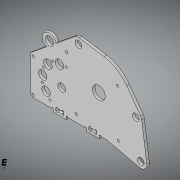
# Autodesk Inventor part: 新型４アームフレーム新
Saved by Autodesk Inventor 2019 (Build 230136000, 136)
## iProperties
Created: 2019-09-30
Part Number: 新型４アームフレーム新
Material: 一般
Document SubType Name: Modeling
Designer: tanjihayato
Density: 1 g/cm^3
Appearance: 既定
Author: tanjihayato
Autodesk Inventor part; units mm, degrees
ref_plane "YZ Plane" through (0, 0, 0) normal (1, 0, 0) x (0, 1, 0)
ref_plane "XZ Plane" through (0, 0, 0) normal (0, 1, 0) x (-1, 0, 0)
ref_plane "XY Plane" through (0, 0, 0) normal (0, 0, 1) x (1, 0, 0)
sketch "スケッチ1" plane through (0, 0, 0) normal (0, 0, 1) x (1, 0, 0)
  circle A0 centre (-22.9427, -32.8237) radius 14
  circle A1 centre (5.0573, -32.8237) radius 14
  line L0 (-174.7493, -46.8237) -> (173.7138, -46.8237)
  line L1 (-168.9427, 85.6498) -> (-168.9427, -143.3841)
  line L2 (181.0573, 70.1234) -> (181.0573, -176.3692)
  line L3 (-68.9427, 93.6608) -> (-68.9427, -144.401)
  circle A2 centre (-138.9427, -9.8237) radius 4.5
  circle A3 centre (-32.6636, -19.9769) radius 20.05
  circle A4 centre (-50.9427, -32.8237) radius 14
  circle A5 centre (-48.8152, -4.5402) radius 14
  circle A6 centre (-32.6636, -19.9769) radius 9.0359
  circle A7 centre (10.5145, -3.7237) radius 37.1
  circle A8 centre (-48.8152, -4.5402) radius 2.292
  circle A9 centre (-48.8152, -4.5402) radius 2.792
  circle A10 centre (10.5145, -3.7237) radius 39.1
  circle A11 centre (53.6032, -6.8237) radius 33.1
  circle A12 centre (53.6032, -6.8237) radius 35.1
  line L4 (-120.6193, -91.8237) -> (100.4081, -91.8237)
  circle A13 centre (10.5145, -3.7237) radius 10.1
  circle A14 centre (10.5145, -3.7237) radius 12.1
  circle A15 centre (-32.6636, -19.9769) radius 20.55
  line L5 (53.6032, -6.8237) -> (32.39, 14.3895)
  line L6 (53.6032, -6.8237) -> (97.5006, -47.7262)
  line L7 (97.5006, -47.7262) -> (57.2048, -10.293)
  line L8 (57.2048, -10.293) -> (32.39, 14.3895)
  circle A16 centre (32.39, 14.3895) radius 1.5
  circle A17 centre (32.39, 14.3895) radius 4.5
  circle A18 centre (-54.9427, -18.301) radius 14
  circle A19 centre (-35.3456, 2.2036) radius 14
  circle A20 centre (-50.9427, -32.8237) radius 5
  circle A21 centre (-54.9427, -18.301) radius 5
  circle A22 centre (-48.8152, -4.5402) radius 5
  circle A23 centre (-35.3456, 2.2036) radius 5
  circle A24 centre (-32.6636, -19.9769) radius 22.342 construction
  line L9 (-43.4189, -43.5289) -> (-55.5427, -26.2785) construction
  line L10 (-55.5427, -26.2785) -> (-54.3426, -10.3236) construction
  line L11 (-54.3426, -10.3236) -> (-43.2878, 1.2432) construction
  line L12 (-43.2878, 1.2432) -> (-22.1495, 3.7992) construction
  circle A25 centre (-35.3456, 2.2036) radius 8
  circle A26 centre (-48.8152, -4.5402) radius 8
  circle A27 centre (-54.9427, -18.301) radius 8
  circle A28 centre (-50.9427, -32.8237) radius 8
  circle A29 centre (-46.3426, -39.3689) radius 1.3
  circle A30 centre (-55.5427, -26.2785) radius 1.3
  circle A31 centre (-54.3426, -10.3236) radius 1.3
  circle A32 centre (-43.2878, 1.2432) radius 1.3
  circle A33 centre (-27.4035, 3.1639) radius 1.3
  circle A34 centre (-35.3456, 2.2036) radius 5.5 construction
  line L13 (-89.4402, -42.8237) -> (131.6872, -42.8237)
  circle A35 centre (53.6032, -6.8237) radius 3
  circle A36 centre (97.5006, -47.7262) radius 7.025
  circle A37 centre (97.5006, -47.7262) radius 10.025
  circle A38 centre (57.2048, -10.293) radius 5
  line L14 (60.2589, -6.3341) -> (103.6241, -39.7887)
  line L15 (90.035, -54.4169) -> (53.4813, -13.63)
  point P0 (0, 0)
  point P1 (0, 0)
  point P2 (0, 0)
  dimension "d0" = 350
  dimension "d1" = 100
  dimension "d2" = 30
  dimension "d3" = 40.1
  dimension "d4" = 28
  dimension "d5" = 28
  dimension "d6" = 22.342
  dimension "d7" = 22.342
  dimension "d9" = 74.2
  dimension "d10" = 0.5
  dimension "d11" = 2
  dimension "d13" = 66.2
  dimension "d14" = 2
  dimension "d15" = 45
  dimension "d16" = 85
  dimension "d17" = 2
  dimension "d18" = 0.5
  dimension "d19" = 30
  dimension "d20" = 60
  dimension "d21" = 55
  dimension "d22" = 35
  dimension "d23" = 45
  dimension "d24" = 3
  dimension "d25" = 3
  dimension "d26" = 28
  dimension "d27" = 28
  dimension "d28" = 22.342
  dimension "d29" = 22.342
  dimension "d30" = 10
  dimension "d31" = 10
  dimension "d32" = 10
  dimension "d33" = 10
  dimension "d34" = 3
  dimension "d35" = 3
  dimension "d36" = 3
  dimension "d37" = 3
  dimension "d38" = 2.6
  dimension "d39" = 2.6
  dimension "d40" = 2.6
  dimension "d41" = 2.6
  dimension "d42" = 2.6
  dimension "d43" = 11
  dimension "d44" = 20.2
  dimension "d45" = 4
  dimension "d46" = 6
  dimension "d48" = 46.1359
  dimension "d60" = 14.05
  dimension "d61" = 3
  dimension "d62" = 10
  constraints: 38 centre point, 32 end point, 14 coincident, 12 point on circle, 10 tangent, 7 point on line, 4 vertical, 3 horizontal, 2 midpoint, 1 equal radius, 9 other
  measures "d0" distance between parallel lines of L2 L1
  measures "d1" distance between parallel lines of L1 L3
  measures "d2" distance from line of L1 A2.centre
  measures "d3" diameter of A3
  measures "d4" diameter of A4
  measures "d5" diameter of A5
  measures "d6" distance of A5.centre A3.centre
  measures "d7" distance of A4.centre A3.centre
  measures "d9" diameter of A7
  measures "d10" radial gap between concentric circles of A8 A9
  measures "d11" radial gap between concentric circles of A7 A10
  measures "d13" diameter of A11
  measures "d14" radial gap between concentric circles of A11 A12
  measures "d15" distance between parallel lines of L4 L0
  measures "d16" distance from line of L4 L5.start
  measures "d17" radial gap between concentric circles of A13 A14
  measures "d18" radial gap between concentric circles of A3 A15
  measures "d19" distance of L5.start L5.end
  measures "d20" distance of L5.start L6.end
  measures "d21" distance of L6.end L7.end
  measures "d22" distance of L7.end L5.end
  measures "d23" angle of L0 L5
  measures "d24" diameter of A16
  measures "d25" radial gap between concentric circles of A16 A17
  measures "d26" diameter of A18
  measures "d27" diameter of A19
  measures "d28" distance of A3.centre A19.centre
  measures "d29" distance of A3.centre A18.centre
  measures "d30" diameter of A20
  measures "d31" diameter of A21
  measures "d32" diameter of A22
  measures "d33" diameter of A23
  measures "d34" radial gap between concentric circles of A23 A25
  measures "d35" radial gap between concentric circles of A22 A26
  measures "d36" radial gap between concentric circles of A21 A27
  measures "d37" radial gap between concentric circles of A20 A28
  measures "d38" diameter of A29
  measures "d39" diameter of A30
  measures "d40" diameter of A31
  measures "d41" diameter of A32
  measures "d42" diameter of A33
  measures "d43" diameter of A34
  measures "d44" diameter of A13
  measures "d45" distance between parallel lines of L0 L13
  measures "d46" diameter of A35
  measures "d48" distance of A3.centre A13.centre
  measures "d60" diameter of A36
  measures "d61" radial gap between concentric circles of A36 A37
  measures "d62" diameter of A38
sketch "スケッチ2" plane through (0, 0, 0) normal (0, 0, 1) x (1, 0, 0)
  circle A0 centre (-47.2698, 19.7966) radius 5.025
  circle A1 centre (-64.0841, -20.5754) radius 1.5
  line L0 (-60.2999, -17.1214) -> (-60.1004, -16.784)
  arc A2 (-59.1969, -16.2937) -> (-60.1004, -16.784) centre (-59.2396, -17.2928) ccw
  arc A3 (-59.1969, -16.2937) -> (-55.0576, -13.6829) centre (-59.0136, -11.9976) ccw
  arc A4 (-54.227, -13.0788) -> (-55.0576, -13.6829) centre (-54.1376, -14.0748) ccw
  arc A5 (-54.227, -13.0788) -> (-49.4577, -10.9346) centre (-54.9427, -5.1109) ccw
  arc A6 (-48.2633, -10.8017) -> (-49.4577, -10.9346) centre (-48.7721, -11.6625) ccw
  line L1 (-48.2633, -10.8017) -> (-43.4665, -13.6371)
  arc A7 (-43.0029, -14.7312) -> (-43.4665, -13.6371) centre (-43.9754, -14.498) ccw
  arc A8 (-43.0029, -14.7312) -> (-42.2107, -20.2197) centre (-35.7096, -16.4799) ccw
  arc A9 (-42.346, -21.4001) -> (-42.2107, -20.2197) centre (-43.0775, -20.7183) ccw
  line L2 (-42.346, -21.4001) -> (-46.1452, -25.4763)
  arc A10 (-47.3285, -25.6866) -> (-46.1452, -25.4763) centre (-46.8767, -24.7945) ccw
  arc A11 (-47.3285, -25.6866) -> (-52.5094, -24.9786) centre (-50.9427, -32.8237) ccw
  arc A12 (-53.4769, -24.634) -> (-52.5094, -24.9786) centre (-52.7053, -23.998) ccw
  arc A13 (-53.4769, -24.634) -> (-58.1856, -23.3003) centre (-56.7949, -27.3692) ccw
  arc A14 (-59.1909, -23.0856) -> (-58.1856, -23.3003) centre (-58.509, -22.354) ccw
  line L3 (-59.1909, -23.0856) -> (-59.4776, -22.8183)
  arc A15 (-59.7573, -21.812) -> (-59.4776, -22.8183) centre (-58.7958, -22.0868) ccw
  arc A16 (-59.7573, -21.812) -> (-60.2836, -18.1658) centre (-64.0841, -20.5754) ccw
  arc A17 (-60.2999, -17.1214) -> (-60.2836, -18.1658) centre (-59.439, -17.6303) ccw
  line L4 (-59.6973, -41.892) -> (-56.6977, -39.4479)
  arc A18 (-55.4968, -39.4009) -> (-56.6977, -39.4479) centre (-56.066, -40.2231) ccw
  arc A19 (-55.4968, -39.4009) -> (-49.3759, -40.6688) centre (-50.9427, -32.8237) ccw
  arc A20 (-48.4085, -41.0133) -> (-49.3759, -40.6688) centre (-49.1801, -41.6494) ccw
  arc A21 (-48.4085, -41.0133) -> (-47.3017, -41.966) centre (-45.0905, -38.2782) ccw
  arc A22 (-47.816, -43.8237) -> (-47.3017, -41.966) centre (-47.816, -42.8237) ccw
  line L5 (-47.816, -43.8237) -> (-59.0344, -43.8237)
  arc A23 (-60.0177, -43.0055) -> (-59.0344, -43.8237) centre (-59.0344, -42.8237) ccw
  arc A24 (-60.0177, -43.0055) -> (-60.0433, -42.8775) centre (-64.4427, -43.8237) ccw
  arc A25 (-59.6973, -41.892) -> (-60.0433, -42.8775) centre (-59.0656, -42.6672) ccw
  circle A26 centre (-64.4427, 8.987) radius 1.5
  line L6 (-18.7729, 14.1262) -> (-22.731, 11.1451)
  arc A27 (-23.9329, 11.144) -> (-22.731, 11.1451) centre (-23.3326, 11.9439) ccw
  arc A28 (-23.9329, 11.144) -> (-33.4471, 11.2103) centre (-28.7348, 4.7455) ccw
  arc A29 (-34.4699, 11.1174) -> (-33.4471, 11.2103) centre (-34.0361, 12.0184) ccw
  arc A30 (-34.4699, 11.1174) -> (-39.3039, 10.3536) centre (-36.335, 7.243) ccw
  arc A31 (-40.3065, 10.1269) -> (-39.3039, 10.3536) centre (-39.9943, 11.077) ccw
  line L7 (-40.3065, 10.1269) -> (-40.6789, 10.2493)
  arc A32 (-41.3548, 11.0456) -> (-40.6789, 10.2493) centre (-40.3667, 11.1993) ccw
  arc A33 (-41.3548, 11.0456) -> (-41.5389, 11.7966) centre (-45.8013, 10.3537) ccw
  arc A34 (-40.8249, 13.0896) -> (-41.5389, 11.7966) centre (-40.5917, 12.1172) ccw
  line L8 (-40.8249, 13.0896) -> (-19.5219, 18.1985)
  arc A35 (-18.3194, 16.9804) -> (-19.5219, 18.1985) centre (-19.2887, 17.226) ccw
  arc A36 (-18.3194, 16.9804) -> (-18.3895, 15.0977) centre (-13.9572, 15.8752) ccw
  arc A37 (-18.7729, 14.1262) -> (-18.3895, 15.0977) centre (-19.3745, 14.925) ccw
  circle A38 centre (-13.9572, 15.8752) radius 1.5
  circle A39 centre (21.0458, -37.8866) radius 1.5
  circle A40 centre (30.9378, -6.8237) radius 4.025
  circle A41 centre (-45.0905, -38.2782) radius 1.3
  circle A42 centre (-21.1346, 2.248) radius 1.3
  circle A43 centre (-50.8718, 1.7759) radius 1.3
  arc A44 (-24.4868, -35.136) -> (-25.456, -34.9678) centre (-25.7365, -39.459) ccw
  arc A45 (-26.3109, -34.3678) -> (-25.456, -34.9678) centre (-25.3936, -33.9697) ccw
  line L9 (-26.3109, -34.3678) -> (-31.0992, -23.3351)
  arc A46 (-30.8322, -22.1773) -> (-31.0992, -23.3351) centre (-30.1819, -22.937) ccw
  arc A47 (-30.8322, -22.1773) -> (-28.4693, -18.4362) centre (-35.7096, -16.4799) ccw
  arc A48 (-27.5385, -17.6976) -> (-28.4693, -18.4362) centre (-27.5039, -18.697) ccw
  line L10 (-27.5385, -17.6976) -> (-14.2955, -17.2386)
  arc A49 (-13.2929, -17.9869) -> (-14.2955, -17.2386) centre (-14.2608, -18.238) ccw
  arc A50 (-13.2929, -17.9869) -> (-11.8048, -21.2653) centre (-3.1292, -15.3507) ccw
  arc A51 (-11.9016, -22.5127) -> (-11.8048, -21.2653) centre (-12.6311, -21.8286) ccw
  line L11 (-11.9016, -22.5127) -> (-23.4796, -34.8594)
  arc A52 (-24.4868, -35.136) -> (-23.4796, -34.8594) centre (-24.2091, -34.1754) ccw
  arc A53 (-29.2087, -36.5965) -> (-30.2266, -39.7574) centre (-25.7365, -39.459) ccw
  arc A54 (-31.2244, -40.8237) -> (-30.2266, -39.7574) centre (-31.2244, -39.8237) ccw
  line L12 (-31.2244, -40.8237) -> (-40.0208, -40.8237)
  arc A55 (-40.9773, -39.5321) -> (-40.0208, -40.8237) centre (-40.0208, -39.8237) ccw
  arc A56 (-40.9773, -39.5321) -> (-42.5952, -34.7762) centre (-45.0905, -38.2782) ccw
  arc A57 (-43.0069, -33.8353) -> (-42.5952, -34.7762) centre (-42.0149, -33.9618) ccw
  arc A58 (-43.0069, -33.8353) -> (-44.0772, -28.7169) centre (-50.9427, -32.8237) ccw
  arc A59 (-43.9506, -27.5218) -> (-44.0772, -28.7169) centre (-43.219, -28.2036) ccw
  line L13 (-43.9506, -27.5218) -> (-40.1514, -23.4456)
  arc A60 (-38.9834, -23.2277) -> (-40.1514, -23.4456) centre (-39.4199, -24.1274) ccw
  arc A61 (-38.9834, -23.2277) -> (-34.8793, -23.9338) centre (-35.7096, -16.4799) ccw
  arc A62 (-33.8512, -24.5295) -> (-34.8793, -23.9338) centre (-34.7685, -24.9276) ccw
  line L14 (-33.8512, -24.5295) -> (-29.0629, -35.5622)
  arc A63 (-29.2087, -36.5965) -> (-29.0629, -35.5622) centre (-29.9803, -35.9603) ccw
  circle A64 centre (-25.7365, -39.459) radius 1.5
  line L15 (2.7111, -40.8237) -> (-3.9575, -40.8237)
  line L16 (-3.9575, -40.8237) -> (-3.9575, -42.8237)
  arc A65 (-4.9575, -43.8237) -> (-3.9575, -42.8237) centre (-4.9575, -42.8237) ccw
  line L17 (-4.9575, -43.8237) -> (-21.3858, -43.8237)
  arc A66 (-22.1768, -42.2119) -> (-21.3858, -43.8237) centre (-21.3858, -42.8237) ccw
  arc A67 (-22.1768, -42.2119) -> (-21.5027, -37.9343) centre (-25.7365, -39.459) ccw
  arc A68 (-21.2913, -36.9115) -> (-21.5027, -37.9343) centre (-20.5618, -37.5955) ccw
  line L18 (-21.2913, -36.9115) -> (-9.7133, -24.5648)
  arc A69 (-8.4747, -24.3881) -> (-9.7133, -24.5648) centre (-8.9838, -25.2488) ccw
  arc A70 (-8.4747, -24.3881) -> (-1.928, -25.7817) centre (-3.1292, -15.3507) ccw
  arc A71 (-0.8688, -26.4475) -> (-1.928, -25.7817) centre (-1.8136, -26.7752) ccw
  line L19 (-0.8688, -26.4475) -> (3.6559, -39.4961)
  arc A72 (2.7111, -40.8237) -> (3.6559, -39.4961) centre (2.7111, -39.8237) ccw
  line L20 (-59.0898, 10.8835) -> (-51.3735, 11.4492)
  arc A73 (-50.3006, 10.434) -> (-51.3735, 11.4492) centre (-51.3004, 10.4518) ccw
  arc A74 (-50.3006, 10.434) -> (-49.6018, 7.944) centre (-45.8013, 10.3537) ccw
  arc A75 (-49.5855, 6.8997) -> (-49.6018, 7.944) centre (-50.4463, 7.4085) ccw
  line L21 (-49.5855, 6.8997) -> (-49.785, 6.5622)
  arc A76 (-50.6884, 6.072) -> (-49.785, 6.5622) centre (-50.6458, 7.0711) ccw
  arc A77 (-50.6884, 6.072) -> (-54.8278, 3.4611) centre (-50.8718, 1.7759) ccw
  arc A78 (-55.6583, 2.8571) -> (-54.8278, 3.4611) centre (-55.7478, 3.853) ccw
  arc A79 (-55.6583, 2.8571) -> (-57.3945, 2.5042) centre (-54.9427, -5.1109) ccw
  arc A80 (-58.5302, 2.8972) -> (-57.3945, 2.5042) centre (-57.7009, 3.456) ccw
  line L22 (-58.5302, 2.8972) -> (-60.4611, 5.7626)
  arc A81 (-60.5065, 6.8061) -> (-60.4611, 5.7626) centre (-59.6318, 6.3214) ccw
  arc A82 (-60.5065, 6.8061) -> (-60.0032, 9.7227) centre (-64.4427, 8.987) ccw
  arc A83 (-59.0898, 10.8835) -> (-60.0032, 9.7227) centre (-59.0167, 9.8861) ccw
  line L23 (-41.6154, 7.3992) -> (-41.243, 7.2769)
  arc A84 (-40.5703, 6.4997) -> (-41.243, 7.2769) centre (-41.5552, 6.3268) ccw
  arc A85 (-40.5703, 6.4997) -> (-37.1316, 3.0174) centre (-36.335, 7.243) ccw
  arc A86 (-36.3633, 2.3359) -> (-37.1316, 3.0174) centre (-37.3169, 2.0347) ccw
  arc A87 (-36.3633, 2.3359) -> (-33.2452, -1.8618) centre (-28.7348, 4.7455) ccw
  arc A88 (-32.8589, -2.9999) -> (-33.2452, -1.8618) centre (-33.809, -2.6878) ccw
  line L24 (-32.8589, -2.9999) -> (-34.5985, -8.2936)
  arc A89 (-35.5675, -8.9812) -> (-34.5985, -8.2936) centre (-35.5485, -7.9814) ccw
  arc A90 (-35.5675, -8.9812) -> (-40.7579, -10.9333) centre (-35.7096, -16.4799) ccw
  arc A91 (-41.9399, -11.0546) -> (-40.7579, -10.9333) centre (-41.431, -10.1938) ccw
  line L25 (-41.9399, -11.0546) -> (-46.7367, -8.2191)
  arc A92 (-47.1961, -7.1086) -> (-46.7367, -8.2191) centre (-46.2278, -7.3583) ccw
  arc A93 (-47.1961, -7.1086) -> (-47.6169, -1.8964) centre (-54.9427, -5.1109) ccw
  arc A94 (-47.4881, -0.8775) -> (-47.6169, -1.8964) centre (-46.7012, -1.4946) ccw
  arc A95 (-47.4881, -0.8775) -> (-47.1963, 4.0077) centre (-50.8718, 1.7759) ccw
  arc A96 (-47.2024, 5.0356) -> (-47.1963, 4.0077) centre (-46.3416, 4.5268) ccw
  line L26 (-47.2024, 5.0356) -> (-47.0029, 5.3731)
  arc A97 (-46.0801, 5.8623) -> (-47.0029, 5.3731) centre (-46.1421, 4.8642) ccw
  arc A98 (-46.0801, 5.8623) -> (-42.6319, 7.1591) centre (-45.8013, 10.3537) ccw
  arc A99 (-41.6154, 7.3992) -> (-42.6319, 7.1591) centre (-41.9276, 6.4492) ccw
  circle A100 centre (-45.8013, 10.3537) radius 1.5
  arc A101 (-63.8052, -16.084) -> (-64.7866, -16.1306) centre (-64.0841, -20.5754) ccw
  arc A102 (-65.9427, -15.1428) -> (-64.7866, -16.1306) centre (-64.9427, -15.1428) ccw
  line L27 (-65.9427, -15.1428) -> (-65.9427, 3.5098)
  arc A103 (-64.8518, 4.5056) -> (-65.9427, 3.5098) centre (-64.9427, 3.5098) ccw
  arc A104 (-64.8518, 4.5056) -> (-63.899, 4.52) centre (-64.4427, 8.987) ccw
  arc A105 (-62.9489, 4.0861) -> (-63.899, 4.52) centre (-63.7782, 3.5273) ccw
  line L28 (-62.9489, 4.0861) -> (-61.0181, 1.2208)
  arc A106 (-61.0802, 0.0205) -> (-61.0181, 1.2208) centre (-61.8474, 0.6619) ccw
  arc A107 (-61.0802, 0.0205) -> (-62.2685, -8.3253) centre (-54.9427, -5.1109) ccw
  arc A108 (-62.3973, -9.3442) -> (-62.2685, -8.3253) centre (-63.1842, -8.7272) ccw
  arc A109 (-62.3973, -9.3442) -> (-62.689, -14.2295) centre (-59.0136, -11.9976) ccw
  arc A110 (-62.683, -15.2574) -> (-62.689, -14.2295) centre (-63.5438, -14.7485) ccw
  line L29 (-62.683, -15.2574) -> (-62.8824, -15.5948)
  arc A111 (-63.8052, -16.084) -> (-62.8824, -15.5948) centre (-63.7433, -15.086) ccw
  arc A112 (-15.9284, 11.83) -> (-14.5765, 11.4181) centre (-13.9572, 15.8752) ccw
  arc A113 (-13.7694, 10.7552) -> (-14.5765, 11.4181) centre (-14.7142, 10.4276) ccw
  line L30 (-13.7694, 10.7552) -> (-8.224, -5.2367)
  arc A114 (-8.6436, -6.4153) -> (-8.224, -5.2367) centre (-9.1688, -5.5643) ccw
  arc A115 (-8.6436, -6.4153) -> (-13.451, -13.4244) centre (-3.1292, -15.3507) ccw
  arc A116 (-14.3994, -14.2404) -> (-13.451, -13.4244) centre (-14.434, -13.241) ccw
  line L31 (-14.3994, -14.2404) -> (-27.6424, -14.6994)
  arc A117 (-28.6221, -14.027) -> (-27.6424, -14.6994) centre (-27.6771, -13.7) ccw
  arc A118 (-28.6221, -14.027) -> (-31.3762, -10.3585) centre (-35.7096, -16.4799) ccw
  arc A119 (-31.7484, -9.2302) -> (-31.3762, -10.3585) centre (-30.7984, -9.5423) ccw
  line L32 (-31.7484, -9.2302) -> (-30.0089, -3.9365)
  arc A120 (-29.0228, -3.2493) -> (-30.0089, -3.9365) centre (-29.0588, -4.2487) ccw
  arc A121 (-29.0228, -3.2493) -> (-24.0225, -1.7194) centre (-28.7348, 4.7455) ccw
  arc A122 (-22.9997, -1.6264) -> (-24.0225, -1.7194) centre (-23.4335, -2.5275) ccw
  arc A123 (-22.9997, -1.6264) -> (-20.338, 6.4736) centre (-21.1346, 2.248) ccw
  arc A124 (-21.1063, 7.1551) -> (-20.338, 6.4736) centre (-20.1528, 7.4563) ccw
  arc A125 (-21.1063, 7.1551) -> (-21.2591, 7.5939) centre (-28.7348, 4.7455) ccw
  arc A126 (-20.9262, 8.7487) -> (-21.2591, 7.5939) centre (-20.3246, 7.9499) ccw
  line L33 (-20.9262, 8.7487) -> (-16.968, 11.7298)
  arc A127 (-15.9284, 11.83) -> (-16.968, 11.7298) centre (-16.3664, 10.931) ccw
  arc A128 (-62.6274, -39.7061) -> (-64.8518, -39.3423) centre (-64.4427, -43.8237) ccw
  arc A129 (-65.9427, -38.3465) -> (-64.8518, -39.3423) centre (-64.9427, -38.3465) ccw
  line L34 (-65.9427, -38.3465) -> (-65.9427, -26.008)
  arc A130 (-64.7866, -25.0202) -> (-65.9427, -26.008) centre (-64.9427, -26.008) ccw
  arc A131 (-64.7866, -25.0202) -> (-62.5465, -24.8046) centre (-64.0841, -20.5754) ccw
  arc A132 (-61.523, -25.0129) -> (-62.5465, -24.8046) centre (-62.2049, -25.7444) ccw
  line L35 (-61.523, -25.0129) -> (-61.2363, -25.2801)
  arc A133 (-60.9515, -26.2678) -> (-61.2363, -25.2801) centre (-61.9181, -26.0117) ccw
  arc A134 (-60.9515, -26.2678) -> (-59.2901, -30.8711) centre (-56.7949, -27.3692) ccw
  arc A135 (-58.8785, -31.812) -> (-59.2901, -30.8711) centre (-59.8704, -31.6856) ccw
  arc A136 (-58.8785, -31.812) -> (-58.3042, -35.9554) centre (-50.9427, -32.8237) ccw
  arc A137 (-58.5927, -37.1222) -> (-58.3042, -35.9554) centre (-59.2244, -36.3469) ccw
  line L36 (-58.5927, -37.1222) -> (-61.5923, -39.5663)
  arc A138 (-62.6274, -39.7061) -> (-61.5923, -39.5663) centre (-62.224, -38.791) ccw
  line L37 (7.0584, -40.1513) -> (1.9656, -25.4647)
  arc A139 (2.3852, -24.2861) -> (1.9656, -25.4647) centre (2.9104, -25.137) ccw
  arc A140 (2.3852, -24.2861) -> (4.4427, -22.6251) centre (-3.1292, -15.3507) ccw
  arc A141 (6.0061, -22.7788) -> (4.4427, -22.6251) centre (5.1638, -23.3179) ccw
  arc A142 (6.0061, -22.7788) -> (17.5142, -33.2048) centre (30.9378, -6.8237) ccw
  arc A143 (17.7852, -34.7853) -> (17.5142, -33.2048) centre (17.0607, -34.0961) ccw
  arc A144 (17.7852, -34.7853) -> (16.7058, -36.6975) centre (21.0458, -37.8866) ccw
  arc A145 (11.0425, -40.8237) -> (16.7058, -36.6975) centre (11.2898, -35.2135) ccw
  line L38 (11.0425, -40.8237) -> (8.0032, -40.8237)
  arc A146 (7.0584, -40.1513) -> (8.0032, -40.8237) centre (8.0032, -39.8237) ccw
  circle A147 centre (-64.4427, -43.8237) radius 1.5
  line L39 (-0.9575, -46.8237) -> (-0.9575, -43.8237)
  arc A148 (1.1425, -43.8237) -> (-0.9575, -43.8237) centre (0.0925, -43.8237) ccw
  line L40 (1.1425, -43.8237) -> (5.9425, -43.8237)
  arc A149 (8.0425, -43.8237) -> (5.9425, -43.8237) centre (6.9925, -43.8237) ccw
  line L41 (8.0425, -43.8237) -> (8.0425, -46.8237)
  arc A150 (5.9425, -46.8237) -> (8.0425, -46.8237) centre (6.9925, -46.8237) ccw
  line L42 (5.9425, -46.8237) -> (1.1425, -46.8237)
  arc A151 (-0.9575, -46.8237) -> (1.1425, -46.8237) centre (0.0925, -46.8237) ccw
  circle A152 centre (-3.1292, -15.3507) radius 7.5
  circle A153 centre (-54.9427, -5.1109) radius 5
  circle A154 centre (-35.7096, -16.4799) radius 4.5
  circle A155 centre (-59.0136, -11.9976) radius 1.3
  circle A156 centre (9.7246, 14.3895) radius 1.5
  circle A157 centre (-36.335, 7.243) radius 1.3
  arc A158 (-39.4427, -46.8237) -> (-37.3427, -46.8237) centre (-38.3927, -46.8237) ccw
  line L43 (-39.4427, -46.8237) -> (-39.4427, -43.8237)
  arc A159 (-37.3427, -43.8237) -> (-39.4427, -43.8237) centre (-38.3927, -43.8237) ccw
  line L44 (-37.3427, -43.8237) -> (-32.5427, -43.8237)
  arc A160 (-30.4427, -43.8237) -> (-32.5427, -43.8237) centre (-31.4927, -43.8237) ccw
  line L45 (-30.4427, -46.8237) -> (-30.4427, -43.8237)
  arc A161 (-32.5427, -46.8237) -> (-30.4427, -46.8237) centre (-31.4927, -46.8237) ccw
  line L46 (-32.5427, -46.8237) -> (-37.3427, -46.8237)
  circle A162 centre (-56.7949, -27.3692) radius 1.3
  circle A163 centre (-28.7348, 4.7455) radius 5
  circle A164 centre (-50.9427, -32.8237) radius 5
  circle A165 centre (40.0583, -39.6814) radius 4
  circle A166 centre (23.1152, 26.3669) radius 4
  line L47 (-56.4345, 14.0862) -> (-64.7717, 13.475)
  arc A167 (-64.7717, 13.475) -> (-68.9427, 8.987) centre (-64.4427, 8.987) ccw
  line L48 (-68.9427, 8.987) -> (-68.9427, -43.8237)
  arc A168 (-68.9427, -43.8237) -> (-67.7968, -46.8237) centre (-64.4427, -43.8237) ccw
  line L49 (-67.7968, -46.8237) -> (-44.5427, -46.8237)
  arc A169 (-42.4427, -46.8237) -> (-44.5427, -46.8237) centre (-43.4927, -46.8237) ccw
  line L50 (-42.4427, -46.8237) -> (-42.4427, -49.8237)
  line L51 (-42.4427, -49.8237) -> (-27.4427, -49.8237)
  line L52 (-27.4427, -49.8237) -> (-27.4427, -46.8237)
  arc A170 (-25.3427, -46.8237) -> (-27.4427, -46.8237) centre (-26.3927, -46.8237) ccw
  line L53 (-25.3427, -46.8237) -> (-6.0575, -46.8237)
  arc A171 (-3.9575, -46.8237) -> (-6.0575, -46.8237) centre (-5.0075, -46.8237) ccw
  line L54 (-3.9575, -46.8237) -> (-3.9575, -49.8237)
  line L55 (-3.9575, -49.8237) -> (11.0425, -49.8237)
  line L56 (11.0425, -49.8237) -> (11.0425, -46.8237)
  arc A172 (13.1312, -46.6704) -> (11.0425, -46.8237) centre (12.0925, -46.8237) ccw
  line L57 (13.1312, -46.6704) -> (35.5383, -45.0264)
  arc A173 (35.5383, -45.0264) -> (46.1969, -36.3172) centre (40.0583, -39.6814) ccw
  arc A174 (51.7353, -27.8861) -> (46.1969, -36.3172) centre (68.6944, -45.0614) ccw
  arc A175 (51.7353, -27.8861) -> (45.9909, 18.6629) centre (30.9378, -6.8237) ccw
  line L58 (45.9909, 18.6629) -> (29.8762, 28.1807)
  arc A176 (29.8762, 28.1807) -> (17.1853, 30.0866) centre (23.1152, 26.3669) ccw
  line L59 (17.1853, 30.0866) -> (-36.8037, 17.139)
  arc A177 (-39.2651, 19.2261) -> (-36.8037, 17.139) centre (-37.2702, 19.0839) ccw
  arc A178 (-39.2651, 19.2261) -> (-54.7232, 16.8221) centre (-47.2698, 19.7966) ccw
  arc A179 (-56.4345, 14.0862) -> (-54.7232, 16.8221) centre (-56.5808, 16.0808) ccw
  point P0 (0, 0)
  point P1 (0, 0)
  point P2 (0, 0)
  constraints: 314 point on circle, 180 centre point, 120 end point
sketch "スケッチ3" plane through (0, 0, 0) normal (0, 0, 1) x (1, 0, 0)
  line L0 (-3.9575, -49.8237) -> (11.0425, -49.8237) projected
  line L1 (11.0425, -49.8237) -> (11.0425, -46.8237) projected
  arc A0 (13.1312, -46.6704) -> (11.0425, -46.8237) centre (12.0925, -46.8237) ccw projected
  line L2 (-3.9575, -46.8237) -> (-3.9575, -49.8237) projected
  arc A1 (-3.9575, -46.8237) -> (-6.0575, -46.8237) centre (-5.0075, -46.8237) ccw projected
  arc A2 (-25.3427, -46.8237) -> (-27.4427, -46.8237) centre (-26.3927, -46.8237) ccw projected
  line L3 (-27.4427, -49.8237) -> (-27.4427, -46.8237) projected
  line L4 (-42.4427, -49.8237) -> (-27.4427, -49.8237) projected
  line L5 (-42.4427, -46.8237) -> (-42.4427, -49.8237) projected
  arc A3 (-42.4427, -46.8237) -> (-44.5427, -46.8237) centre (-43.4927, -46.8237) ccw projected
  circle A4 centre (53.6032, -6.8237) radius 35.1 construction
  circle A5 centre (10.5145, -3.7237) radius 39.1 construction
  circle A6 centre (-35.3456, 2.2036) radius 5 projected
  circle A7 centre (-27.4035, 3.1639) radius 1.3 projected
  circle A8 centre (-43.2878, 1.2432) radius 1.3 projected
  circle A9 centre (-48.8152, -4.5402) radius 5 projected
  circle A10 centre (-54.3426, -10.3236) radius 1.3 projected
  circle A11 centre (-54.9427, -18.301) radius 5 projected
  circle A12 centre (-55.5427, -26.2785) radius 1.3 projected
  circle A13 centre (-50.9427, -32.8237) radius 5 projected
  circle A14 centre (-46.3426, -39.3689) radius 1.3 projected
  circle A15 centre (-32.6636, -19.9769) radius 20.55 construction
  circle A16 centre (32.39, 14.3895) radius 1.5 projected
  circle A17 centre (-32.6636, -19.9769) radius 4.5
  circle A18 centre (10.5145, -3.7237) radius 7.5
  circle A19 centre (53.6032, -6.8237) radius 4.025
  line L6 (-68.9427, 93.6608) -> (-68.9427, -144.401) projected
  line L7 (-44.5427, -46.8237) -> (-65.9427, -46.8237)
  line L8 (-25.3427, -46.8237) -> (-6.0575, -46.8237)
  circle A20 centre (-47.2698, 19.7966) radius 5.025 projected
  arc A21 (-39.3675, 21.1943) -> (-50.246, 12.3439) centre (-47.2698, 19.7966) ccw
  arc A22 (42.988, 19.8025) -> (16.6575, 35.903) centre (10.5145, -3.7237) ccw
  circle A23 centre (-35.3456, 2.2036) radius 14 construction
  line L9 (-68.9427, -2.8673) -> (-68.9427, -43.8237)
  circle A24 centre (-13.2119, 33.4498) radius 4
  arc A25 (-12.1396, 40.3671) -> (-17.6296, 38.8797) centre (-13.2119, 33.4498) ccw
  circle A26 centre (53.6032, -6.8237) radius 7.025
  circle A27 centre (59.4446, -48.5165) radius 4
  line L10 (-12.1396, 40.3671) -> (16.6575, 35.903)
  line L11 (42.988, 19.8025) -> (59.2921, -2.7022)
  arc A28 (57.8936, -55.3425) -> (66.3775, -47.5493) centre (59.4446, -48.5165) ccw
  line L12 (60.5608, -5.8531) -> (66.3775, -47.5493)
  line L13 (19.7272, -46.6704) -> (57.8936, -55.3425)
  circle A29 centre (-65.8016, -5.2211) radius 3 construction
  circle A30 centre (-48.8152, -4.5402) radius 14 construction
  circle A31 centre (-54.9427, -18.301) radius 14 construction
  circle A32 centre (33.3605, -40.8589) radius 4.5 construction
  circle A33 centre (33.3605, -40.8589) radius 1.5
  arc A34 (-68.9427, -43.8237) -> (-65.9427, -46.8237) centre (-65.9427, -43.8237) ccw
  arc A35 (-32.5427, -46.8237) -> (-30.4427, -46.8237) centre (-31.4927, -46.8237) ccw projected
  line L14 (-32.5427, -46.8237) -> (-37.3427, -46.8237) projected
  arc A36 (-39.4427, -46.8237) -> (-37.3427, -46.8237) centre (-38.3927, -46.8237) ccw projected
  line L15 (-39.4427, -46.8237) -> (-39.4427, -43.8237) projected
  arc A37 (-37.3427, -43.8237) -> (-39.4427, -43.8237) centre (-38.3927, -43.8237) ccw projected
  line L16 (-37.3427, -43.8237) -> (-32.5427, -43.8237) projected
  arc A38 (-30.4427, -43.8237) -> (-32.5427, -43.8237) centre (-31.4927, -43.8237) ccw projected
  arc A39 (5.9425, -46.8237) -> (8.0425, -46.8237) centre (6.9925, -46.8237) ccw projected
  line L17 (5.9425, -46.8237) -> (1.1425, -46.8237) projected
  arc A40 (-0.9575, -46.8237) -> (1.1425, -46.8237) centre (0.0925, -46.8237) ccw projected
  line L18 (-0.9575, -46.8237) -> (-0.9575, -43.8237) projected
  arc A41 (1.1425, -43.8237) -> (-0.9575, -43.8237) centre (0.0925, -43.8237) ccw projected
  line L19 (1.1425, -43.8237) -> (5.9425, -43.8237) projected
  arc A42 (8.0425, -43.8237) -> (5.9425, -43.8237) centre (6.9925, -43.8237) ccw projected
  line L20 (8.0425, -43.8237) -> (8.0425, -46.8237) projected
  line L21 (-30.4427, -46.8237) -> (-30.4427, -43.8237) projected
  line L22 (13.1312, -46.6704) -> (19.7272, -46.6704)
  circle A43 centre (-65.8016, -5.2211) radius 1.5
  circle A44 centre (-65.9427, -43.8237) radius 1.5
  line L23 (-17.6296, 38.8797) -> (-39.3675, 21.1943)
  line L24 (-50.246, 12.3439) -> (-68.9427, -2.8673)
  circle A45 centre (-15.7921, -38.4932) radius 1.5
  circle A46 centre (-15.7921, -38.4932) radius 4.5 construction
  circle A47 centre (-26.8994, 18.6629) radius 1.5
  circle A48 centre (-26.8994, 18.6629) radius 4.5 construction
  point P0 (0, 0)
  dimension "d49" = 9
  dimension "d50" = 15
  dimension "d51" = 8.05
  dimension "d52" = 3
  dimension "d53" = 1
  dimension "d54" = 28
  dimension "d55" = 8
  dimension "d56" = 3
  dimension "d57" = 3
  dimension "d58" = 8
  dimension "d59" = 3
  dimension "d63" = 6
  dimension "d64" = 9
  dimension "d65" = 3
  dimension "d66" = 6
  dimension "d67" = 3
  dimension "d68" = 3
  dimension "d69" = 3
  dimension "d70" = 9
  dimension "d71" = 3
  dimension "d72" = 9
  constraints: 23 tangent, 21 centre point, 20 end point, 12 point on circle, 9 coincident, 2 collinear, 2 horizontal, 1 point on line
  measures "d49" diameter of A17
  measures "d50" diameter of A18
  measures "d51" diameter of A19
  measures "d52" radial gap between concentric circles of A20 A21
  measures "d53" radial gap between concentric circles of A5 A22
  measures "d54" diameter of A23
  measures "d55" diameter of A24
  measures "d56" radial gap between concentric circles of A24 A25
  measures "d57" radial gap between concentric circles of A19 A26
  measures "d58" diameter of A27
  measures "d59" radial gap between concentric circles of A27 A28
  measures "d63" diameter of A29
  measures "d64" diameter of A32
  measures "d65" diameter of A33
  measures "d66" diameter of A34
  measures "d67" diameter of A43
  measures "d68" diameter of A44
  measures "d69" diameter of A45
  measures "d70" diameter of A46
  measures "d71" diameter of A47
  measures "d72" diameter of A48
extrude "押し出し1" add sketch "スケッチ3" along normal blind 3
equation "\"d7\" = d6"
equation "\"d28\" = d6"
equation "\"d29\" = d6"
